Autodesk Inventor part; units mm, degrees
(part 2 of 2)
sketch "Эскиз6" plane through (0, 0, 0) normal (0, -1, 0) x (0.7730105, 0, 0.6343933)
  circle A0 centre (0, 0) radius 36.8469 projected
  arc A1 (-24.3345, 27.6681) -> (24.3345, 27.6681) centre (0, 84.2847) ccw
  arc A2 (24.3345, -27.6681) -> (-24.3345, -27.6681) centre (0, -84.2847) ccw
  arc A3 (28.8177, 22.9616) -> (28.8177, -22.9616) centre (59.4541, 0) ccw
  line L0 (24.3345, 27.6681) -> (-24.3345, 27.6681) construction
  line L1 (-24.3345, -27.6681) -> (24.3345, -27.6681) construction
  line L2 (8.168, 17.66) -> (-36.8469, 17.66) construction
  line L3 (28.8177, 22.9616) -> (28.8177, -22.9616) construction
  line L4 (8.168, -17.913) -> (8.168, 17.66) construction
  line L5 (24.3345, 27.6681) -> (28.8177, 22.9616) construction
  line L6 (28.8177, 22.9616) -> (27.4535, 21.6622) construction
  point P0 (0, 22.66)
  point P1 (21.168, 0)
  dimension "d13" = 5
  dimension "d15" = 6.5
  dimension "d16" = 13
  constraints: 14 point on circle, 10 end point, 3 centre point, 3 parallel, 2 perpendicular, 1 equal radius
  measures "d13" distance from line of L2 point (0, 22.66)
  measures "d15" distance from line of L6 L0.start
  measures "d16" distance from line of L4 point (21.168, 0)
sketch "Эскиз8" plane through (0, 0, 0) normal (0, -1, 0) x (0.7730105, 0, 0.6343933)
  circle A0 centre (31.3386, 14.384) radius 3.05 construction
  circle A1 centre (7.9937, 33.5427) radius 3.05 construction
  circle A2 centre (-7.9937, -33.5427) radius 3.05 construction
  circle A3 centre (-31.3386, -14.384) radius 3.05 construction
  circle A4 centre (0, 0) radius 36.8469 projected
  circle A5 centre (0, 0) radius 44.0469
  line L0 (27.9044, 34.0805) -> (27.9817, 34.017) projected
  circle A6 centre (0, 0) radius 45.3132
  arc A7 (26.8105, 36.5306) -> (23.49, 38.7493) centre (0, 0) ccw projected
  circle A8 centre (7.9937, 33.5427) radius 1.55
  circle A9 centre (31.3386, 14.384) radius 1.55
  circle A10 centre (-7.9937, -33.5427) radius 1.55
  circle A11 centre (-31.3386, -14.384) radius 1.55
  point P0 (27.9431, 34.0487)
  point P1 (25.1747, 37.6766)
  dimension "d37" = 3.1
  constraints: 6 coincident, 4 centre point, 3 equal radius, 1 midpoint, 1 point on circle, 6 other
  measures "d37" diameter of A8
extrude "Выдавливание4" add sketch "Эскиз8" against normal up to surface (2 mm away)
sketch "Эскиз16" plane through (0, 2, 0) normal (0, 1, 0) x (0.0980171, 0, 0.9951847)
  point P0 (0, 0)
extrude "Выдавливание10" cut sketch "Эскиз42" against normal blind 10 contours L36 A105 L37 A104 | L38 A106 L39 A107
